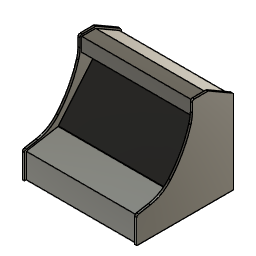
Tetris v2 (Autodesk Fusion 360 design; units mm, degrees)
Autodesk Fusion 360 part; units mm, degrees
sketch "LED dispaly" plane through (0, 0, 0) normal (0, 0, 1) x (1, 0, 0)
  line L0 (-99.8242, 44.7455) -> (51.1758, 44.7455) construction
  line L1 (-107.8242, 54.2455) -> (210.1758, 54.2455)
  line L2 (-107.8242, 54.2455) -> (-107.8242, -103.7545)
  line L3 (-107.8242, -103.7545) -> (210.1758, -103.7545)
  line L4 (210.1758, -103.7545) -> (210.1758, 54.2455)
  line L5 (-99.8242, 44.7455) -> (-99.8242, -94.2545) construction
  circle A0 centre (-99.8242, 44.7455) radius 1.7
  circle A1 centre (-99.8242, -94.2545) radius 1.7
  line L6 (51.1758, 44.7455) -> (51.1758, 23.1533) construction
  line L7 (-24.3242, 44.7455) -> (-24.3242, 22.2115) construction
  circle A2 centre (51.1758, 44.7455) radius 1.7
  circle A3 centre (51.1758, -94.2545) radius 1.7
  circle A4 centre (202.1758, 44.7455) radius 1.7
  circle A5 centre (202.1758, -94.2545) radius 1.7
  line L8 (-99.8242, 44.7455) -> (-99.8242, 54.2455) construction
  line L9 (-99.8242, -94.2545) -> (-99.8242, -103.7545) construction
  line L10 (-99.8242, 44.7455) -> (-107.8242, 44.7455) construction
  line L11 (202.1758, 44.7455) -> (210.1758, 44.7455) construction
  dimension "d1" = 151
  dimension "d2" = 318
  dimension "d3" = 158
  dimension "d4" = 139
  dimension "d5" = 3.4
  dimension "d7" = 3.4
  constraint horizontal L0
  constraint horizontal L1
  constraint perpendicular L1 L2
  constraint perpendicular L2 L3
  constraint perpendicular L1 L4
  constraint perpendicular L0 L5
  constraint coincident L0.start L5.start
  constraint coincident L5.end A1.centre
  constraint perpendicular L0 L6
  constraint midpoint L0 L7.start
  constraint perpendicular L0 L7
  constraint symmetric A0 L7 A2
  constraint symmetric A1 L7 A3
  constraint symmetric A0 L6 A4
  constraint symmetric A1 L6 A5
  constraint coincident L1 L8.end
  constraint perpendicular L1 L8
  constraint coincident L3 L9.end
  constraint perpendicular L3 L9
  constraint coincident L2 L10.end
  constraint perpendicular L2 L10
  constraint coincident A4.centre L11.start
  constraint coincident L4 L11.end
  constraint perpendicular L4 L11
  constraint equal L10 L11
  constraint equal L8 L9
  measures "d1" distance of L0.start L0.end
  measures "d2" distance of L1.start L1.end
  measures "d3" distance of L1.start L2.end
  measures "d4" distance of L0.start L5.end
  measures "d5" diameter of A0
  measures "d7" diameter of A1
extrude "Extrude1" add sketch "LED dispaly" against normal blind 15 makes body 1
extrude "Extrude2" add sketch "LED dispaly" against normal blind 7 contours A0 | A1 | A2 | A3 | A4 | A5 bodies 1
move_body "Move1" bodies 1 to x (1, 0, 0) y (0, 0.642788, 0.766044) z (0, -0.766044, 0.642788) at (0, -48.5531, 74.1224)
ref_plane "WorkPlane1" through (211.1758, -58.7196, 50.3384) normal (1, 0, 0) x (0, -0.642788, -0.766044)
sketch "Cabinet" plane through (211.1758, 0, 0) normal (1, 0, 0) x (0, 1, 0)
  line L0 (-13.6847, 115.6768) -> (-115.2452, -5.3582)
  line L1 (-115.2452, -5.3582) -> (-103.7545, -15)
  line L2 (-103.7545, -15) -> (-2.1941, 106.035)
  line L3 (-2.1941, 106.035) -> (-13.6847, 115.6768)
  line L4 (-47.514, 145.3683) -> (-47.514, 185.3683)
  line L5 (-47.514, 185.3683) -> (-7.514, 185.3683)
  line L6 (-7.514, 185.3683) -> (61.7681, 145.3683)
  line L7 (-2.1941, 106.035) -> (-1.5513, 106.8011)
  line L8 (-1.5513, 106.8011) -> (-47.514, 145.3683)
  line L9 (61.7681, -93.965) -> (-208.2319, -93.965)
  line L10 (-208.2319, -93.965) -> (-208.2319, -22.407)
  line L11 (-115.2452, -5.3582) -> (-115.888, -6.1242)
  line L12 (-115.888, -6.1242) -> (-104.3973, -15.766)
  line L13 (-115.888, -6.1242) -> (-208.2319, -22.407)
  line L14 (-103.7545, -15) -> (-104.3973, -15.766)
  line L15 (-2.1941, 106.035) -> (61.7681, 106.035) construction
  line L16 (61.7681, 106.035) -> (61.7681, -93.965)
  line L17 (61.7681, 145.3683) -> (61.7681, 106.035)
  line L18 (0.8701, 103.4639) -> (4.084, 107.2941)
  line L19 (4.084, 107.2941) -> (-43.514, 147.2336)
  line L20 (-43.514, 147.2336) -> (-43.514, 181.3683)
  line L21 (-43.514, 181.3683) -> (-8.5858, 181.3683)
  line L22 (-8.5858, 181.3683) -> (57.7681, 143.0589)
  line L23 (57.7681, 143.0589) -> (57.7681, 106.035)
  line L24 (57.7681, 106.035) -> (57.7681, -89.965)
  line L25 (57.7681, -89.965) -> (-204.2319, -89.965)
  line L26 (-204.2319, -89.965) -> (-204.2319, -25.7634)
  line L27 (-117.0303, -10.3874) -> (-204.2319, -25.7634)
  line L28 (-117.0303, -10.3874) -> (-103.9043, -21.4014)
  line L29 (-100.6903, -17.5712) -> (-103.9043, -21.4014)
  line L30 (-103.7545, -15) -> (-100.6903, -17.5712)
  line L31 (-2.1941, 106.035) -> (0.8701, 103.4639)
  line L32 (57.7681, 143.0589) -> (61.7681, 145.3683)
  line L33 (57.7681, -89.965) -> (57.7681, -93.965)
  line L34 (-13.6847, 115.6768) -> (-13.042, 116.4429)
  arc A0 (-140.5082, -10.4654) -> (-47.514, 145.3683) centre (-339.5616, 213.9844) ccw
  arc A1 (-142.7746, -5.7879) -> (-52.514, 145.9503) centre (-339.5616, 213.9844) ccw
  line L35 (-52.514, 145.9503) -> (-52.514, 190.3683)
  line L36 (-52.514, 190.3683) -> (-6.1742, 190.3683)
  line L37 (-6.1742, 190.3683) -> (66.7681, 148.2551)
  line L38 (66.7681, 148.2551) -> (66.7681, 106.035)
  line L39 (66.7681, 106.035) -> (66.7681, -98.965)
  line L40 (66.7681, -98.965) -> (-213.2319, -98.965)
  line L41 (-213.2319, -98.965) -> (-213.2319, -18.2115)
  line L42 (-142.7746, -5.7879) -> (-213.2319, -18.2115)
  line L43 (-208.2319, -93.965) -> (-213.2319, -93.965)
  line L44 (61.7681, -93.965) -> (66.7681, -93.965)
  dimension "d15" = 40
  dimension "d16" = 40
  dimension "d17" = 80
  dimension "d20" = 1
  dimension "d21" = 60
  dimension "d22" = 270
  dimension "d23" = 1
  dimension "d25" = 130
  dimension "d26" = 150
  dimension "d27" = 200
  dimension "d28" = 4
  dimension "d36" = 300
  dimension "d38" = 25
  dimension "d39" = -5
  constraint vertical L4
  constraint perpendicular L4 L5
  constraint coincident L2.end L3.start
  constraint perpendicular L3 L7
  constraint perpendicular L2 L8
  constraint perpendicular L9 L10
  constraint coincident L0.end L1.start
  constraint perpendicular L1 L11
  constraint perpendicular L2 L12
  constraint coincident L10 L13.end
  constraint coincident L1.end L2.start
  constraint coincident L12 L14.end
  constraint perpendicular L12 L14
  constraint perpendicular L15 L16
  constraint perpendicular L9 L16
  constraint vertical L17
  constraint parallel L16 L17
  constraint perpendicular L29 L30
  constraint perpendicular L7 L31
  constraint coincident L9 L33.end
  constraint perpendicular L9 L33
  constraint coincident L0.start L3.end
  constraint coincident L8 L34.end
  constraint perpendicular L8 L34
  constraint coincident L13 A0.start
  constraint coincident L41 L43.end
  constraint perpendicular L41 L43
  constraint coincident L39 L44.end
  constraint perpendicular L39 L44
  measures "d15" distance of L4.end L4.start
  measures "d16" distance of L4.end L5.end
  measures "d17" distance of L5.end L6.end
  measures "d20" distance of L2.end L7.end
  measures "d21" distance of L7.end L4.start
  measures "d22" distance of L9.start L9.end
  measures "d23" distance of L0.end L11.end
  measures "d25" angle of L12 L13
  measures "d26" angle of L5 L6
  measures "d27" distance of L9.start L15.end
  measures "d36" radius of A0
  measures "d38" distance of L11.end A0.start
ref_plane "WorkPlane2" through (51.6758, -58.7196, 50.3384) normal (-1, 0, 0) x (0, 0.642788, 0.766044)
extrude "Extrude3" add sketch "Cabinet" along normal blind 6 separate body contours L0 L1 L2 L3 | L3 L7 L8 L34 | L0 L8 L11 L13 L34 A0 | L1 L11 L12 L14 | L2 L18 L19 L20 L21 L22 L23 L24 L25 L26 L27 L28 L29 L30 L31 | L4 L5 L6 L7 L8 L18 L19 L20 L21 L22 L31 L32 | L9 L10 L12 L13 L14 L25 L26 L27 L28 L29 L30 L33 | L4 L5 L6 L10 L13 L16 L17 A0 A1 L35 L36 L37 L38 L39 L41 L42 L43 L44 | L9 L16 L17 L23 L24 L32 L33 makes body 2
fillet "Fillet1" radius 6 4 edges at (214.1758, -52.514, 190.3683) (214.1758, 66.7681, 148.2551) (214.1758, -213.2319, -18.2115) (214.1758, -6.1742, 190.3683) on bodies 2
fillet "Fillet1" radius 100 2 edges at (214.1758, -52.514, 145.9503) (214.1758, -142.7746, -5.7879) on bodies 2
mirror "Mirror1" about plane through (51.6758, -58.7196, 50.3384) normal (-1, 0, 0) of bodies 2 makes body 3
extrude "Extrude4" add sketch "Cabinet" against normal up to surface (319 mm away) contours L4 L5 L6 L7 L8 L18 L19 L20 L21 L22 L31 L32 | L9 L10 L12 L13 L14 L25 L26 L27 L28 L29 L30 L33 bodies 2 3
equation "d5 = m3"
equation "m3 = 3.4 mm"
equation "d7 = m3"
